Autodesk Fusion 360 part; units mm, degrees
(part 2 of 2)
sketch "Sketch3 (1)" plane through (0, 0, 3) normal (0, 0, 1) x (-1, 0, 0)
  circle A0 centre (-55.1926, -65.2253) radius 1.75
  circle A1 centre (-118.1555, -65.2253) radius 1.75
  circle A2 centre (-5.0937, -5.0744) radius 1.75
  circle A3 centre (-127.1555, -65.2253) radius 4.65
  circle A4 centre (-5.0937, -77.7497) radius 1.75
  circle A5 centre (-168.257, -5.0744) radius 1.75
  circle A6 centre (-168.257, -77.7497) radius 1.75
  circle A7 centre (-46.1926, -65.2253) radius 4.65
  line L0 (-173.257, -82.7497) -> (-0.0937, -82.7497)
  line L1 (-0.0937, -82.7497) -> (-0.0937, -0.0744)
  line L2 (-0.0937, -0.0744) -> (-173.257, -0.0744)
  line L3 (-173.257, -0.0744) -> (-173.257, -82.7497)
  line L4 (-152.7305, -72.2256) -> (-152.7305, -73.2256)
  line L5 (-152.7305, -73.2256) -> (-158.7305, -73.2256)
  line L6 (-158.7305, -73.2256) -> (-158.7305, -72.2256)
  line L7 (-158.7305, -72.2256) -> (-162.731, -72.2256)
  line L8 (-162.731, -72.2256) -> (-162.731, -58.2249)
  line L9 (-162.731, -58.2249) -> (-158.7305, -58.2249)
  line L10 (-158.7305, -58.2249) -> (-158.7305, -57.2249)
  line L11 (-158.7305, -57.2249) -> (-152.7305, -57.2249)
  line L12 (-152.7305, -57.2249) -> (-152.7305, -58.2249)
  line L13 (-152.7305, -58.2249) -> (-148.73, -58.2249)
  line L14 (-148.73, -58.2249) -> (-148.73, -72.2256)
  line L15 (-148.73, -72.2256) -> (-152.7305, -72.2256)
  line L16 (-101.5807, -58.2249) -> (-101.5807, -57.2249)
  line L17 (-101.5807, -57.2249) -> (-95.5807, -57.2249)
  line L18 (-95.5807, -57.2249) -> (-95.5807, -58.2249)
  line L19 (-95.5807, -58.2249) -> (-91.5804, -58.2249)
  line L20 (-91.5804, -58.2249) -> (-91.5804, -72.2256)
  line L21 (-91.5804, -72.2256) -> (-95.5807, -72.2256)
  line L22 (-95.5807, -72.2256) -> (-95.5807, -73.2256)
  line L23 (-95.5807, -73.2256) -> (-101.5807, -73.2256)
  line L24 (-101.5807, -73.2256) -> (-101.5807, -72.2256)
  line L25 (-101.5807, -72.2256) -> (-105.581, -72.2256)
  line L26 (-105.581, -72.2256) -> (-105.581, -58.2249)
  line L27 (-105.581, -58.2249) -> (-101.5807, -58.2249)
  line L28 (-58.7189, -44.6492) -> (-58.7189, -43.6492)
  line L29 (-58.7189, -43.6492) -> (-62.7186, -43.6492)
  line L30 (-62.7186, -43.6492) -> (-62.7186, -29.6499)
  line L31 (-62.7186, -29.6499) -> (-58.719, -29.6499)
  line L32 (-58.719, -29.6499) -> (-58.719, -28.6499)
  line L33 (-58.719, -28.6499) -> (-52.7189, -28.6499)
  line L34 (-52.7189, -28.6499) -> (-52.7189, -29.6499)
  line L35 (-52.7189, -29.6499) -> (-48.7193, -29.6499)
  line L36 (-48.7193, -29.6499) -> (-48.7193, -43.6492)
  line L37 (-48.7193, -43.6492) -> (-52.7189, -43.6492)
  line L38 (-52.7189, -43.6492) -> (-52.7189, -44.6492)
  line L39 (-52.7189, -44.6492) -> (-58.7189, -44.6492)
  line L40 (-24.1433, -24.5994) -> (-24.1433, -25.5994)
  line L41 (-24.1433, -25.5994) -> (-30.1433, -25.5994)
  line L42 (-30.1433, -25.5994) -> (-30.1433, -24.5994)
  line L43 (-30.1433, -24.5994) -> (-34.1437, -24.5994)
  line L44 (-34.1437, -24.5994) -> (-34.1437, -10.5999)
  line L45 (-34.1437, -10.5999) -> (-30.1433, -10.5999)
  line L46 (-30.1433, -10.5999) -> (-30.1433, -9.5999)
  line L47 (-30.1433, -9.5999) -> (-24.1433, -9.5999)
  line L48 (-24.1433, -9.5999) -> (-24.1433, -10.5999)
  line L49 (-24.1433, -10.5999) -> (-20.1428, -10.5999)
  line L50 (-20.1428, -10.5999) -> (-20.1428, -24.5994)
  line L51 (-20.1428, -24.5994) -> (-24.1433, -24.5994)
  line L52 (-71.769, -72.2256) -> (-71.769, -73.2256)
  line L53 (-71.769, -73.2256) -> (-77.769, -73.2256)
  line L54 (-77.769, -73.2256) -> (-77.769, -72.2256)
  line L55 (-77.769, -72.2256) -> (-81.7686, -72.2256)
  line L56 (-81.7686, -72.2256) -> (-81.7686, -58.2249)
  line L57 (-81.7686, -58.2249) -> (-77.769, -58.2249)
  line L58 (-77.769, -58.2249) -> (-77.769, -57.2249)
  line L59 (-77.769, -57.2249) -> (-71.769, -57.2249)
  line L60 (-71.769, -57.2249) -> (-71.769, -58.2249)
  line L61 (-71.769, -58.2249) -> (-67.7693, -58.2249)
  line L62 (-67.7693, -58.2249) -> (-67.7693, -72.2256)
  line L63 (-67.7693, -72.2256) -> (-71.769, -72.2256)
  line L64 (-158.7305, -44.6492) -> (-158.7305, -43.6492)
  line L65 (-158.7305, -43.6492) -> (-162.731, -43.6492)
  line L66 (-162.731, -43.6492) -> (-162.731, -29.6499)
  line L67 (-162.731, -29.6499) -> (-158.7305, -29.6499)
  line L68 (-158.7305, -29.6499) -> (-158.7305, -28.6499)
  line L69 (-158.7305, -28.6499) -> (-152.7305, -28.6499)
  line L70 (-152.7305, -28.6499) -> (-152.7305, -29.6499)
  line L71 (-152.7305, -29.6499) -> (-148.73, -29.6499)
  line L72 (-148.73, -29.6499) -> (-148.73, -43.6492)
  line L73 (-148.73, -43.6492) -> (-152.7305, -43.6492)
  line L74 (-152.7305, -43.6492) -> (-152.7305, -44.6492)
  line L75 (-152.7305, -44.6492) -> (-158.7305, -44.6492)
  line L76 (-149.2055, -25.5994) -> (-149.2055, -24.5994)
  line L77 (-149.2055, -24.5994) -> (-153.206, -24.5994)
  line L78 (-153.206, -24.5994) -> (-153.206, -10.5999)
  line L79 (-153.206, -10.5999) -> (-149.2055, -10.5999)
  line L80 (-149.2055, -10.5999) -> (-149.2055, -9.5999)
  line L81 (-149.2055, -9.5999) -> (-143.2055, -9.5999)
  line L82 (-143.2055, -9.5999) -> (-143.2055, -10.5999)
  line L83 (-143.2055, -10.5999) -> (-139.205, -10.5999)
  line L84 (-139.205, -10.5999) -> (-139.205, -24.5994)
  line L85 (-139.205, -24.5994) -> (-143.2055, -24.5994)
  line L86 (-143.2055, -24.5994) -> (-143.2055, -25.5994)
  line L87 (-143.2055, -25.5994) -> (-149.2055, -25.5994)
  line L88 (-62.2426, -9.5999) -> (-62.2426, -10.5999)
  line L89 (-62.2426, -10.5999) -> (-58.2429, -10.5999)
  line L90 (-58.2429, -10.5999) -> (-58.2429, -24.5994)
  line L91 (-58.2429, -24.5994) -> (-62.2426, -24.5994)
  line L92 (-62.2426, -24.5994) -> (-62.2426, -25.5994)
  line L93 (-62.2426, -25.5994) -> (-68.2425, -25.5994)
  line L94 (-68.2425, -25.5994) -> (-68.2425, -24.5994)
  line L95 (-68.2425, -24.5994) -> (-72.2422, -24.5994)
  line L96 (-72.2422, -24.5994) -> (-72.2422, -10.5999)
  line L97 (-72.2422, -10.5999) -> (-68.2426, -10.5999)
  line L98 (-68.2426, -10.5999) -> (-68.2426, -9.5999)
  line L99 (-68.2426, -9.5999) -> (-62.2426, -9.5999)
  line L100 (-114.6305, -28.6499) -> (-114.6305, -29.6499)
  line L101 (-114.6305, -29.6499) -> (-110.63, -29.6499)
  line L102 (-110.63, -29.6499) -> (-110.63, -43.6492)
  line L103 (-110.63, -43.6492) -> (-114.6305, -43.6492)
  line L104 (-114.6305, -43.6492) -> (-114.6305, -44.6492)
  line L105 (-114.6305, -44.6492) -> (-120.6305, -44.6492)
  line L106 (-120.6305, -44.6492) -> (-120.6305, -43.6492)
  line L107 (-120.6305, -43.6492) -> (-124.631, -43.6492)
  line L108 (-124.631, -43.6492) -> (-124.631, -29.6499)
  line L109 (-124.631, -29.6499) -> (-120.6305, -29.6499)
  line L110 (-120.6305, -29.6499) -> (-120.6305, -28.6499)
  line L111 (-120.6305, -28.6499) -> (-114.6305, -28.6499)
  line L112 (-111.1055, -25.5994) -> (-111.1055, -24.5994)
  line L113 (-111.1055, -24.5994) -> (-115.106, -24.5994)
  line L114 (-115.106, -24.5994) -> (-115.106, -10.5999)
  line L115 (-115.106, -10.5999) -> (-111.1055, -10.5999)
  line L116 (-111.1055, -10.5999) -> (-111.1055, -9.5999)
  line L117 (-111.1055, -9.5999) -> (-105.1055, -9.5999)
  line L118 (-105.1055, -9.5999) -> (-105.1055, -10.5999)
  line L119 (-105.1055, -10.5999) -> (-101.105, -10.5999)
  line L120 (-101.105, -10.5999) -> (-101.105, -24.5994)
  line L121 (-101.105, -24.5994) -> (-105.1055, -24.5994)
  line L122 (-105.1055, -24.5994) -> (-105.1055, -25.5994)
  line L123 (-105.1055, -25.5994) -> (-111.1055, -25.5994)
  line L124 (-14.6183, -43.6492) -> (-14.6183, -44.6492)
  line L125 (-14.6183, -44.6492) -> (-20.6183, -44.6492)
  line L126 (-20.6183, -44.6492) -> (-20.6183, -43.6492)
  line L127 (-20.6183, -43.6492) -> (-24.6187, -43.6492)
  line L128 (-24.6187, -43.6492) -> (-24.6187, -29.6499)
  line L129 (-24.6187, -29.6499) -> (-20.6183, -29.6499)
  line L130 (-20.6183, -29.6499) -> (-20.6183, -28.6499)
  line L131 (-20.6183, -28.6499) -> (-14.6183, -28.6499)
  line L132 (-14.6183, -28.6499) -> (-14.6183, -29.6499)
  line L133 (-14.6183, -29.6499) -> (-10.6178, -29.6499)
  line L134 (-10.6178, -29.6499) -> (-10.6178, -43.6492)
  line L135 (-10.6178, -43.6492) -> (-14.6183, -43.6492)
  line L136 (-130.1555, -25.5994) -> (-130.1555, -24.5994)
  line L137 (-130.1555, -24.5994) -> (-134.156, -24.5994)
  line L138 (-134.156, -24.5994) -> (-134.156, -10.5999)
  line L139 (-134.156, -10.5999) -> (-130.1555, -10.5999)
  line L140 (-130.1555, -10.5999) -> (-130.1555, -9.5999)
  line L141 (-130.1555, -9.5999) -> (-124.1555, -9.5999)
  line L142 (-124.1555, -9.5999) -> (-124.1555, -10.5999)
  line L143 (-124.1555, -10.5999) -> (-120.155, -10.5999)
  line L144 (-120.155, -10.5999) -> (-120.155, -24.5994)
  line L145 (-120.155, -24.5994) -> (-124.1555, -24.5994)
  line L146 (-124.1555, -24.5994) -> (-124.1555, -25.5994)
  line L147 (-124.1555, -25.5994) -> (-130.1555, -25.5994)
  line L148 (-133.6805, -28.6499) -> (-133.6805, -29.6499)
  line L149 (-133.6805, -29.6499) -> (-129.68, -29.6499)
  line L150 (-129.68, -29.6499) -> (-129.68, -43.6492)
  line L151 (-129.68, -43.6492) -> (-133.6805, -43.6492)
  line L152 (-133.6805, -43.6492) -> (-133.6805, -44.6492)
  line L153 (-133.6805, -44.6492) -> (-139.6805, -44.6492)
  line L154 (-139.6805, -44.6492) -> (-139.6805, -43.6492)
  line L155 (-139.6805, -43.6492) -> (-143.681, -43.6492)
  line L156 (-143.681, -43.6492) -> (-143.681, -29.6499)
  line L157 (-143.681, -29.6499) -> (-139.6805, -29.6499)
  line L158 (-139.6805, -29.6499) -> (-139.6805, -28.6499)
  line L159 (-139.6805, -28.6499) -> (-133.6805, -28.6499)
  line L160 (-49.1926, -25.5994) -> (-49.1926, -24.5994)
  line L161 (-49.1926, -24.5994) -> (-53.1922, -24.5994)
  line L162 (-53.1922, -24.5994) -> (-53.1922, -10.5999)
  line L163 (-53.1922, -10.5999) -> (-49.1926, -10.5999)
  line L164 (-49.1926, -10.5999) -> (-49.1926, -9.5999)
  line L165 (-49.1926, -9.5999) -> (-43.1926, -9.5999)
  line L166 (-43.1926, -9.5999) -> (-43.1926, -10.5999)
  line L167 (-43.1926, -10.5999) -> (-39.1929, -10.5999)
  line L168 (-39.1929, -10.5999) -> (-39.1929, -24.5994)
  line L169 (-39.1929, -24.5994) -> (-43.1926, -24.5994)
  line L170 (-43.1926, -24.5994) -> (-43.1926, -25.5994)
  line L171 (-43.1926, -25.5994) -> (-49.1926, -25.5994)
  line L172 (-39.6689, -44.6492) -> (-39.6689, -43.6492)
  line L173 (-39.6689, -43.6492) -> (-43.6686, -43.6492)
  line L174 (-43.6686, -43.6492) -> (-43.6686, -29.6499)
  line L175 (-43.6686, -29.6499) -> (-39.6689, -29.6499)
  line L176 (-39.6689, -29.6499) -> (-39.6689, -28.6499)
  line L177 (-39.6689, -28.6499) -> (-33.6689, -28.6499)
  line L178 (-33.6689, -28.6499) -> (-33.6689, -29.6499)
  line L179 (-33.6689, -29.6499) -> (-29.6692, -29.6499)
  line L180 (-29.6692, -29.6499) -> (-29.6692, -43.6492)
  line L181 (-29.6692, -43.6492) -> (-33.6689, -43.6492)
  line L182 (-33.6689, -43.6492) -> (-33.6689, -44.6492)
  line L183 (-33.6689, -44.6492) -> (-39.6689, -44.6492)
  line L184 (-0.0937, -67.7497) -> (-32.0937, -67.7497)
  line L185 (-32.0937, -67.7497) -> (-32.0937, -56.7497)
  line L186 (-32.0937, -56.7497) -> (-0.0937, -56.7497)
  line L187 (-0.0937, -56.7497) -> (-0.0937, -67.7497)
  dimension "d91" = 32
  dimension "d92" = 11
  dimension "d93" = 15
  constraint horizontal L184
  constraint vertical L185
  constraint horizontal L186
  constraint vertical L187
  constraint coincident L1 L184.start
  measures "d91" distance of L184.start L184.end
  measures "d92" distance of L184.start L186.end
  measures "d93" distance of L0 L184
extrude "Extrude2'" add sketch "Sketch3 (1)" along normal blind 1.5 contours L1 L184 L185 L186 L187
fillet "Fillet1" radius 3 4 edges at (173.257, 0.0744, 1.5) (173.257, 82.7497, 1.5) (0.0937, 0.0744, 1.5) (0.0937, 82.7497, 1.5)
move_body "Move1" bodies 1 to x (-1, 0, 0) y (0, 1, 0) z (0, 0, -1) at (167.7679, 0, 6)
